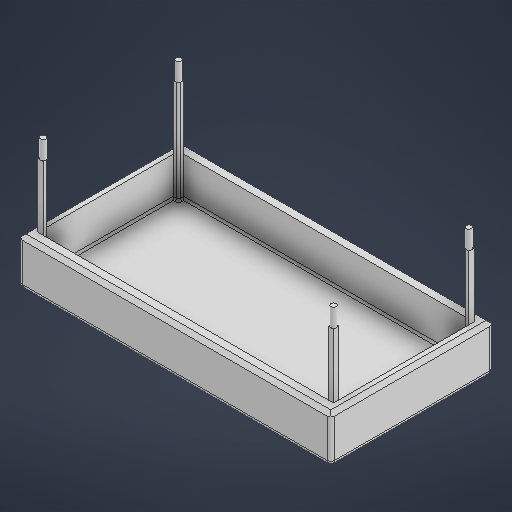
# Autodesk Inventor part: Buggy_Body
Saved by Autodesk Inventor 2026.1 (Build 301233000, 233)
## iProperties
Created: 2026-02-09
Part Number: Buggy_Body
Material: Generic
Document SubType Name: Modeling
Designer: dm2166
Density: 1 g/cm^3
Appearance: Default
Author: dm2166
Autodesk Inventor part; units mm, degrees
ref_plane "YZ Plane" through (0, 0, 0) normal (1, 0, 0) x (0, 1, 0)
ref_plane "XZ Plane" through (0, 0, 0) normal (0, 1, 0) x (-1, 0, 0)
ref_plane "XY Plane" through (0, 0, 0) normal (0, 0, 1) x (1, 0, 0)
sketch "Sketch1" plane through (0, 0, 0) normal (0, 1, 0) x (-1, 0, 0)
  line L0 (-85.5, -44.5) -> (85.5, -44.5)
  line L1 (85.5, -44.5) -> (85.5, 44.5)
  line L2 (85.5, 44.5) -> (-85.5, 44.5)
  line L3 (-85.5, 44.5) -> (-85.5, -44.5)
  line L4 (-85.5, -44.5) -> (85.5, 44.5) construction
  line L5 (85.5, -44.5) -> (-85.5, 44.5) construction
  line L6 (-81, -38.5) -> (81, -38.5)
  line L7 (81, -38.5) -> (81, 38.5)
  line L8 (81, 38.5) -> (-81, 38.5)
  line L9 (-81, 38.5) -> (-81, -38.5)
  line L10 (-81, -38.5) -> (81, 38.5) construction
  line L11 (81, -38.5) -> (-81, 38.5) construction
  line L12 (81, 38.5) -> (79.55, 38.5)
  line L13 (81, 37.05) -> (81, 38.5)
  circle A0 centre (79.55, 37.05) radius 1.45
  circle A1 centre (79.55, -37.05) radius 1.45
  circle A2 centre (-79.55, -37.05) radius 1.45
  circle A3 centre (-79.55, 37.05) radius 1.45
  line L14 (81, 38.5) -> (78.1, 38.5)
  line L15 (78.1, 38.5) -> (78.1, 35.6)
  line L16 (78.1, 35.6) -> (81, 35.6)
  line L17 (81, 35.6) -> (81, 38.5)
  line L18 (81, 38.5) -> (78.1, 35.6) construction
  line L19 (78.1, 38.5) -> (81, 35.6) construction
  line L20 (81, -35.6) -> (78.1, -35.6)
  line L21 (78.1, -35.6) -> (78.1, -38.5)
  line L22 (78.1, -38.5) -> (81, -38.5)
  line L23 (81, -38.5) -> (81, -35.6)
  line L24 (81, -35.6) -> (78.1, -38.5) construction
  line L25 (78.1, -35.6) -> (81, -38.5) construction
  line L26 (-78.1, -35.6) -> (-81, -35.6)
  line L27 (-81, -35.6) -> (-81, -38.5)
  line L28 (-81, -38.5) -> (-78.1, -38.5)
  line L29 (-78.1, -38.5) -> (-78.1, -35.6)
  line L30 (-78.1, -35.6) -> (-81, -38.5) construction
  line L31 (-81, -35.6) -> (-78.1, -38.5) construction
  line L32 (-78.1, 38.5) -> (-81, 38.5)
  line L33 (-81, 38.5) -> (-81, 35.6)
  line L34 (-81, 35.6) -> (-78.1, 35.6)
  line L35 (-78.1, 35.6) -> (-78.1, 38.5)
  line L36 (-78.1, 38.5) -> (-81, 35.6) construction
  line L37 (-81, 38.5) -> (-78.1, 35.6) construction
  point P0 (0, 0)
  point P1 (-79.55, 38.5)
  point P2 (-81, 37.05)
  point P3 (-81, -37.05)
  point P4 (-79.55, -38.5)
  point P5 (79.55, -38.5)
  point P6 (81, -37.05)
  dimension "d0" = 171
  dimension "d1" = 89
  dimension "d2" = 162
  dimension "d3" = 77
  dimension "d7" = 2.9
  dimension "d8" = 2.9
  dimension "d9" = 2.9
  dimension "d10" = 2.9
  constraints: 76 end point, 12 midpoint, 12 parallel, 8 tangent, 7 horizontal, 6 perpendicular, 5 point on line, 4 centre point
  measures "d0" distance of L2.end L1.end
  measures "d1" distance of L1.end L0.end
  measures "d2" distance of L8.end L7.end
  measures "d3" distance of L7.end L6.end
  measures "d7" diameter of A0
  measures "d8" diameter of A1
  measures "d9" diameter of A2
  measures "d10" diameter of A3
extrude "Extrusion1" add sketch "Sketch1" along normal blind 70 contours A2 | A1 | A3 | A0
extrude "Extrusion2" add sketch "Sketch1" along normal blind 4 contours L29 L26 L9 L34 L35 L8 L15 L16 L7 L20 L21 L6 | L6 A2 L29 | L21 A1 L6 | A2 L26 L29 | L21 L20 A1 | L9 L26 A2 | A1 L20 L7 | L9 A3 L34 | L16 A0 L7 | A3 L35 L34 | L16 L15 A0 | L8 L35 A3 | A0 L15 L8
extrude "Extrusion3" add sketch "Sketch1" along normal blind 25
extrude "Extrusion4" add sketch "Sketch1" along normal blind 60 contours L6 L9 A2
extrude "Extrusion5" add sketch "Sketch1" along normal blind 60 contours L6 A2 L29 | L6 L9 A2 | A2 | A2 L26 L29 | L9 L26 A2
extrude "Extrusion6" add sketch "Sketch1" along normal blind 60 contours L9 A3 L34 | L9 L8 A3 | A3 | A3 L35 L34 | L8 L35 A3
extrude "Extrusion7" add sketch "Sketch1" along normal blind 60 contours L16 A0 L7 | A0 L8 L7 | A0 | L16 L15 A0 | A0 L15 L8
extrude "Extrusion8" add sketch "Sketch1" along normal blind 60 contours L21 A1 L6 | A1 L7 L6 | A1 | L21 L20 A1 | A1 L20 L7
fillet "Fillet1" radius 1 1 edges at (-78.1, 32, -35.6)
fillet "Fillet2" radius 1 1 edges at (-78.1, 32, 35.6)
fillet "Fillet3" radius 1 1 edges at (78.1, 32, 35.6)
fillet "Fillet4" radius 1 1 edges at (78.1, 32, -35.6)
fillet "Fillet5" radius 1 16 edges at (-81, 4, 0) (-78.1, 4, -37.55) (-80.05, 4, -35.6) (-78.3929, 4, -35.8929) (0, 4, -38.5) (0, 4, 38.5) (-78.3929, 4, 35.8929) (-80.05, 4, 35.6) (-78.1, 4, 37.55) (80.05, 4, -35.6) (78.1, 4, -37.55) (78.3929, 4, -35.8929) (81, 4, 0) (78.3929, 4, 35.8929) (80.05, 4, 35.6) (78.1, 4, 37.55)
chamfer "Chamfer1" distance 2 angle 45 4 edges at (0, 25, 44.5) (85.5, 25, 0) (0, 25, -44.5) (-85.5, 25, 0)
fillet "Fillet6" radius 2 1 edges at (85.5, 11.5, 44.5)
fillet "Fillet7" radius 2 1 edges at (85.5, 11.5, -44.5)
fillet "Fillet8" radius 2 1 edges at (-85.5, 11.5, 44.5)
fillet "Fillet9" radius 2 1 edges at (-85.5, 11.5, -44.5)
fillet "Fillet10" radius 2 4 edges at (-85.5, 0, 0) (0, 0, 44.5) (85.5, 0, 0) (0, 0, -44.5)
body "Solid1"
